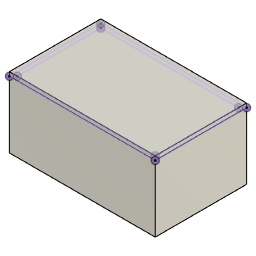
Dual SSR Relay Casing v5 (Autodesk Fusion 360 design; units mm, degrees)
Autodesk Fusion 360 part; units mm, degrees
sketch "Base" plane through (0, 0, 0) normal (0, 0, 1) x (1, 0, 0)
  line L0 (29.2, 18.3) -> (-29.2, 18.3)
  line L1 (-29.2, 18.3) -> (-29.2, -18.3)
  line L2 (-29.2, -18.3) -> (29.2, -18.3)
  line L3 (29.2, -18.3) -> (29.2, 18.3)
  line L4 (29.2, 18.3) -> (-29.2, -18.3) construction
  line L5 (-29.2, 18.3) -> (29.2, -18.3) construction
  point P0 (-29.2, 0)
  dimension "d1" = 58.4
  dimension "d2" = 36.6
  constraint horizontal L0
  constraint perpendicular L0 L1
  constraint parallel L0 L2
  constraint parallel L1 L3
  constraint coincident L4 origin
  constraint coincident L5 origin
  constraint midpoint L1 P0
  measures "d1" distance of L1.end L2.end
  measures "d2" distance of L0.end L1.end
extrude "Extrusion1" add sketch "Base" along normal blind 28.2 makes body 1
shell "Schale1" thickness 1.6 removed faces 0 bodies 1
ref_plane "Arbeitsebene1" through (-27.6, -16.7, 1.6) normal (0, 0, -1) x (-1, 0, 0)
sketch "Skizze3" plane through (-27.6, -16.7, 1.6) normal (0, 0, -1) x (1, 0, 0)
  line L0 (0, 0) -> (55.2, 0)
  line L1 (0, -33.4) -> (0, 0)
  circle A0 centre (2.6, -2.6) radius 2.6
  line L2 (55.2, -33.4) -> (0, -33.4)
  circle A1 centre (2.6, -30.8) radius 2.6
  line L3 (55.2, 0) -> (55.2, -33.4)
  circle A2 centre (52.6, -30.8) radius 2.6
  circle A3 centre (52.6, -2.6) radius 2.6
  circle A4 centre (2.6, -2.6) radius 1.5
  circle A5 centre (2.6, -30.8) radius 1.5
  circle A6 centre (52.6, -30.8) radius 1.5
  circle A7 centre (52.6, -2.6) radius 1.5
  dimension "d7" = 2.6
  dimension "d8" = 2.6
  dimension "d9" = 2.6
  dimension "d10" = 2.6
  dimension "d19" = 3
  dimension "d20" = 3
  dimension "d21" = 3
  dimension "d22" = 3
  constraint tangent L0 A0
  constraint tangent L1 A0
  constraint tangent L2 A1
  constraint tangent L1 A1
  constraint tangent L2 A2
  constraint tangent L3 A2
  constraint tangent L3 A3
  constraint tangent L0 A3
  constraint concentric A0 A4
  constraint concentric A1 A5
  constraint concentric A2 A6
  constraint concentric A3 A7
  measures "d7" radius of A0
  measures "d8" radius of A1
  measures "d9" radius of A2
  measures "d10" radius of A3
  measures "d19" diameter of A4
  measures "d20" diameter of A5
  measures "d21" diameter of A6
  measures "d22" diameter of A7
extrude "Extrusion2" add sketch "Skizze3" against normal blind 2 contours A0 | A3 | A1 | A2 bodies 1
sketch "Hole" plane through (-29.2, 0, 0) normal (-1, 0, 0) x (0, -1, 0)
  line L0 (-18.3, 0) -> (18.3, 0)
  line L1 (18.3, 0) -> (18.3, 28.2)
  line L2 (18.3, 28.2) -> (-18.3, 28.2)
  line L3 (-18.3, 28.2) -> (-18.3, 0)
  line L4 (-11.2, 17.7) -> (11.2, 17.7)
  line L5 (11.2, 17.7) -> (11.2, 5.4)
  line L6 (11.2, 5.4) -> (-11.2, 5.4)
  line L7 (-11.2, 5.4) -> (-11.2, 17.7)
  line L8 (14.1, 1.6) -> (16.7, 1.6)
  line L9 (-14.1, 1.6) -> (14.1, 1.6)
  line L10 (-16.7, 1.6) -> (-14.1, 1.6)
  point P0 (0, 5.4)
  dimension "d13" = 22.4
  dimension "d14" = 12.3
  constraint horizontal L4
  constraint vertical L5
  constraint horizontal L6
  constraint vertical L7
  constraint midpoint L6 P0
  measures "d13" distance of L4.start L4.end
  measures "d14" distance of L4.start L6.end
extrude "Extrusion3" cut sketch "Hole" against normal blind 1.6 contours L4 L5 L6 L7 bodies 1
ref_plane "Arbeitsebene2" through (0, 0, 26.6) normal (0, 0, 1) x (1, 0, 0)
split "Teilen1" by plane through (0, 0, 26.6) normal (0, 0, 1) bodies 1 makes body 2 at (-9.7333, -6.1, 28.2)
sketch "Skizze6" plane through (0, 0, 26.6) normal (0, 0, 1) x (1, 0, 0)
  line L0 (27.6, -16.7) -> (-27.6, -16.7)
  line L1 (-27.6, -16.7) -> (-27.6, 16.7)
  line L2 (-27.6, 16.7) -> (27.6, 16.7)
  line L3 (27.6, 16.7) -> (27.6, -16.7)
  line L4 (-29.2, -18.3) -> (29.2, -18.3)
  line L5 (29.2, -18.3) -> (29.2, 18.3)
  line L6 (29.2, 18.3) -> (-29.2, 18.3)
  line L7 (-29.2, 18.3) -> (-29.2, -18.3)
sketch "Skizze7" plane through (0, 0, 26.6) normal (0, 0, 1) x (1, 0, 0)
  line L0 (29.2, -18.3) -> (-29.2, -18.3)
  line L1 (-29.2, -18.3) -> (-29.2, 18.3)
  line L2 (-29.2, 18.3) -> (29.2, 18.3)
  line L3 (29.2, 18.3) -> (29.2, -18.3)
  line L4 (-27.6, -16.7) -> (27.6, -16.7)
  line L5 (27.6, -16.7) -> (27.6, 16.7)
  line L6 (27.6, 16.7) -> (-27.6, 16.7)
  line L7 (-27.6, 16.7) -> (-27.6, -16.7)
  line L8 (-27.5, 16.6) -> (-27.5, -16.6)
  line L9 (-27.5, -16.6) -> (27.5, -16.6)
  line L10 (27.5, -16.6) -> (27.5, 16.6)
  line L11 (27.5, 16.6) -> (-27.5, 16.6)
  line L12 (27.6, -16.7) -> (-27.6, -16.7)
  line L13 (-27.6, -16.7) -> (-27.6, 16.7)
  line L14 (-27.6, 16.7) -> (27.6, 16.7)
  line L15 (27.6, 16.7) -> (27.6, -16.7)
  line L16 (-29.2, -18.3) -> (29.2, -18.3)
  line L17 (29.2, -18.3) -> (29.2, 18.3)
  line L18 (29.2, 18.3) -> (-29.2, 18.3)
  line L19 (-29.2, 18.3) -> (-29.2, -18.3)
  line L20 (26.5, -15.6) -> (26.5, 15.6)
  line L21 (26.5, 15.6) -> (-26.5, 15.6)
  line L22 (-26.5, 15.6) -> (-26.5, -15.6)
  line L23 (-26.5, -15.6) -> (26.5, -15.6)
  point P0 (-27.6, -16.7)
  dimension "d24" = -0.1
  dimension "d25" = -1.1
extrude "Extrusion4" add sketch "Skizze7" against normal blind 1 contours L8 L9 L10 L11 bodies 2
equation "d1 = 55.2 mm + 2 * wall_thickness"
equation "d2 = 33.4 mm + 2 * wall_thickness"
equation "d3 = 25 mm + 2 * wall_thickness"
equation "d5 = wall_thickness"
equation "wall_thickness = 1.6 mm"
equation "d17 = -wall_thickness"
equation "d23 = -wall_thickness"
named bodies: "Case lower", "Case upper"
